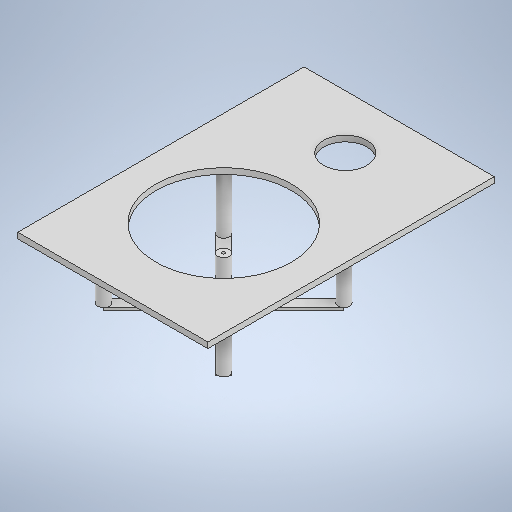
# Autodesk Inventor part: box_cover
Saved by Autodesk Inventor 2025.2 (Build 292293000, 293)
## iProperties
Created: 2025-02-21
Part Number: box_cover
Material: Generic
Document SubType Name: Modeling
Designer: fiste
Density: 1 g/cm^3
Appearance: Default
Author: fiste
Autodesk Inventor part; units mm, degrees
ref_plane "YZ Plane" through (0, 0, 0) normal (1, 0, 0) x (0, 1, 0)
ref_plane "XZ Plane" through (0, 0, 0) normal (0, 1, 0) x (-1, 0, 0)
ref_plane "XY Plane" through (0, 0, 0) normal (0, 0, 1) x (1, 0, 0)
sketch "Sketch1" plane through (0, 0, 0) normal (0, 0, 1) x (1, 0, 0)
  line L0 (0, 0) -> (330, 0)
  line L1 (330, 0) -> (330, 497)
  line L2 (330, 497) -> (0, 497)
  line L3 (0, 497) -> (0, 0)
  dimension "d0" = 330
  dimension "d1" = 497
  constraints: 8 end point, 2 parallel, 1 horizontal, 1 perpendicular
  measures "d0" distance of L2.end L1.end
  measures "d1" distance of L1.end L0.end
extrude "Extrusion1" add sketch "Sketch1" along normal blind 10
sketch "Sketch2" plane through (0, 0, 10) normal (0, 0, 1) x (1, 0, 0)
  circle A0 centre (165, 192.5) radius 117.5
  point P0 (0, 0)
  dimension "d4" = 235
  constraints: 1 centre point
  measures "d4" diameter of A0
extrude "Extrusion2" cut sketch "Sketch2" against normal blind 10
sketch "Sketch3" plane through (0, 0, 10) normal (0, 0, 1) x (1, 0, 0)
  circle A0 centre (165, 403.5) radius 37.5
  point P0 (0, 0)
  dimension "d7" = 75
  constraints: 1 centre point
  measures "d7" diameter of A0
extrude "Extrusion3" cut sketch "Sketch3" against normal blind 10
sketch "Sketch4" plane through (0, 0, 0) normal (0, 0, -1) x (-1, 0, 0)
  circle A0 centre (-269.298, 296.798) radius 10
  circle A1 centre (-165, 192.5) radius 117.5 projected
  circle A2 centre (-269.298, 88.202) radius 10
  circle A3 centre (-60.702, 88.202) radius 10
  circle A4 centre (-60.702, 296.798) radius 10
  point P0 (0, 0)
  dimension "d10" = 20
  dimension "d13" = 360
  constraints: 4 centre point, 1 coincident, 9 other
  measures "d10" diameter of A0
extrude "Extrusion4" add sketch "Sketch4" along normal blind 110 contours A0 | A2 | A3 | A4
sketch "Sketch5" plane through (269.298, 296.798, -110) normal (0, 0, -1) x (-1, 0, 0)
  circle A0 centre (208.596, 0) radius 10 projected
  circle A1 centre (0, -208.596) radius 10 projected
  line L0 (215.6671, -7.0711) -> (7.0711, -215.6671)
  line L1 (201.5249, 7.0711) -> (-7.0711, -201.5249)
  line L2 (7.0711, -215.6671) -> (-7.0711, -201.5249)
  line L3 (201.5249, 7.0711) -> (215.6671, -7.0711)
  circle A2 centre (104.298, -104.298) radius 117.5 projected
  line L4 (7.0711, 7.0711) -> (215.6671, -201.5249)
  line L5 (215.6671, -201.5249) -> (201.5249, -215.6671)
  line L6 (-7.0711, -7.0711) -> (201.5249, -215.6671)
  line L7 (-7.0711, -7.0711) -> (7.0711, 7.0711)
  point P0 (269.298, -296.798)
  point P1 (90.1559, -104.298)
  point P2 (-7.0711, -201.5249)
  point P3 (7.0711, -215.6671)
  point P4 (104.298, -118.4401)
  point P5 (118.4401, -104.298)
  point P6 (215.6671, -7.0711)
  point P7 (104.298, -90.1559)
  point P8 (-7.0711, -201.5249)
  point P9 (7.0711, -215.6671)
  dimension "d21" = 90
  constraints: 16 end point, 1 coincident, 1 perpendicular, 12 other
extrude "Extrusion5" add sketch "Sketch5" along normal blind 5 contours L3 A0 | A0 L0 A2 L1 | A2 L0 L4 L1 | L4 L0 L6 L1 | L1 L6 A2 L4 | A2 L6 L7 L4 | L4 A2 L6 L0 | L6 L0 A2 L1 | L4 L5 L6 A2 | A2 L0 A1 L1 | A1 L2 picked at (207.6691, -4.4554) picked at (2.263, -203.9854)
sketch "Sketch7" plane through (269.298, 296.798, -115) normal (0, 0, -1) x (-1, 0, 0)
  line L0 (90.1559, -104.298) -> (-7.0711, -201.5249) projected
  circle A0 centre (104.5442, -104.298) radius 2.5
  point P0 (269.298, -296.798)
  point P1 (104.298, -118.4401)
  point P2 (104.298, -90.1559)
  dimension "d25" = 5
  constraints: 1 centre point
  measures "d25" diameter of A0
extrude "Extrusion6" add sketch "Sketch7" along normal blind 30
sketch "Sketch8" plane through (269.298, 296.798, -110) normal (0, 0, 1) x (1, 0, 0)
  circle A0 centre (-104.5442, -104.298) radius 2.5 projected
  circle A1 centre (-104.5442, -104.298) radius 2.5
  point P0 (-269.298, -296.798)
  constraints: 2 coincident, 1 centre point, 1 concentric
extrude "Extrusion7" add sketch "Sketch8" along normal blind 40
sketch "Sketch9" plane through (164.7538, 192.5, -70) normal (0, 0, 1) x (1, 0, 0)
  circle A0 centre (0, 0) radius 2.5 projected
  circle A1 centre (0, 0) radius 10
  point P0 (-164.7538, -192.5)
  dimension "d30" = 20
  constraints: 1 centre point, 1 coincident
  measures "d30" diameter of A1
extrude "Extrusion8" add sketch "Sketch9" along normal blind 35
body "Solid1"
